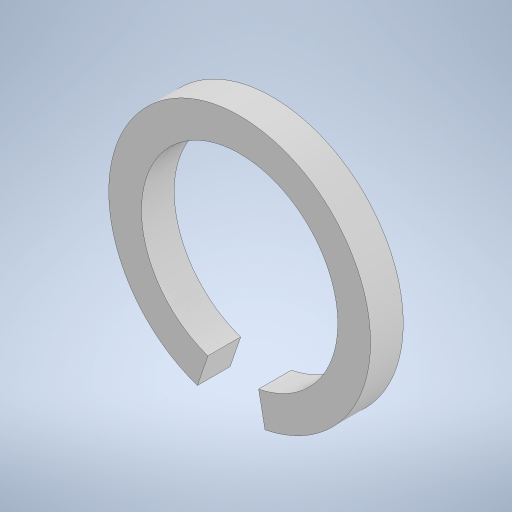
# Autodesk Inventor part: Cring1
Saved by Autodesk Inventor 2023 (Build 270158000, 158)
## iProperties
Created: 2023-05-28
Part Number: Cring1
Material: 一般
Document SubType Name: Modeling
Designer: 310611102
Density: 1 g/cm^3
Appearance: 預設
Author: 310611102
Autodesk Inventor part; units mm, degrees
ref_plane "YZ Plane" through (0, 0, 0) normal (1, 0, 0) x (0, 1, 0)
ref_plane "XZ Plane" through (0, 0, 0) normal (0, 1, 0) x (-1, 0, 0)
ref_plane "XY Plane" through (0, 0, 0) normal (0, 0, 1) x (1, 0, 0)
sketch "Sketch1" plane through (0, 0, 0) normal (0, 0, 1) x (1, 0, 0)
  arc A0 (1.1623, -5.8864) -> (-1.9366, -5.6789) centre (0, 0) ccw
  line L0 (0, 0) -> (-2.7093, -7.9447)
  line L1 (0, 0) -> (1.6067, -8.1374)
  arc A1 (1.5497, -7.8485) -> (-2.5822, -7.5718) centre (0, 0) ccw
  line L2 (-1.9366, -5.6789) -> (-2.5822, -7.5718)
  line L3 (1.1623, -5.8864) -> (1.5497, -7.8485)
  point P0 (1.5497, -7.8485)
  point P1 (-2.5822, -7.5718)
  dimension "d0" = 12
  dimension "d1" = 30
  dimension "d2" = 2
  constraints: 8 end point, 4 point on circle, 2 centre point, 2 point on line, 1 coincident, 1 collinear
  measures "d0" diameter of A0
  measures "d1" angle of L1 L0
  measures "d2" radial gap between concentric circles of A0 A1
extrude "Extrusion1" add sketch "Sketch1" along normal blind 2 contours A0 L0 A1 L1
body "Solid1"
